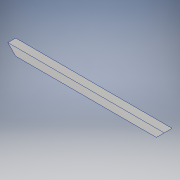
# Autodesk Inventor part: SUP_004_TopConnectorBar
Saved by Autodesk Inventor 2018 (Build 220112000, 112)
## iProperties
Created: 2020-01-26
Part Number: SUP_004_TopConnectorBar
Material: Aluminum 6061
Document SubType Name: Modeling
Designer: user
Mass: 157.364 g
Surface Area: 738.55 cm^2
Volume: 58.2829 cm^3
Density: 2.7 g/cm^3
Appearance: Aluminum - Flat
Author: user
Autodesk Inventor part; units mm, degrees
ref_plane "YZ Plane" through (0, 0, 0) normal (1, 0, 0) x (0, 1, 0)
ref_plane "XZ Plane" through (0, 0, 0) normal (0, 1, 0) x (-1, 0, 0)
ref_plane "XY Plane" through (0, 0, 0) normal (0, 0, 1) x (1, 0, 0)
sketch "Sketch1" plane through (0, 0, 0) normal (1, 0, 0) x (0, 1, 0)
  line L0 (0, 0) -> (25.4, 0)
  line L1 (25.4, 0) -> (25.4, -25.4)
  line L2 (25.4, -25.4) -> (0, -25.4)
  line L3 (0, -25.4) -> (0, 0)
  line L4 (23.8125, -1.5875) -> (1.5875, -1.5875)
  line L5 (1.5875, -1.5875) -> (1.5875, -23.8125)
  line L6 (1.5875, -23.8125) -> (23.8125, -23.8125)
  line L7 (23.8125, -23.8125) -> (23.8125, -1.5875)
  dimension "d0" = 25.4
  dimension "d1" = 25.4
  dimension "d2" = 1.5875
  constraints: 16 end point, 4 parallel, 2 perpendicular, 1 horizontal, 3 other
  measures "d0" distance of L1.end L2.end
  measures "d1" distance of L0.end L1.end
  measures "d2" distance between parallel lines of L0 L4
extrude "Extrusion1" add sketch "Sketch1" along normal mid plane 504.2916
chamfer "Chamfer1" distance 25.4 angle 45 1 edges at (252.1458, 0, -12.7)
chamfer "Chamfer2" distance 25.4 angle 45 1 edges at (-252.1458, 0, -12.7)
body "Solid1"
